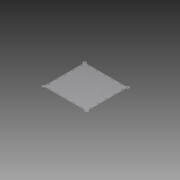
# Autodesk Inventor part: TopPlate2
Saved by Autodesk Inventor 2015 SP1 (Build 190203100, 203)
## iProperties
Created: 2014-08-06
Part Number: TopPlate2
Material: Acrylic, Clear
Document SubType Name: Modeling
Designer: Patrick Camilleri
Density: 1.19 g/cm^3
Appearance: Transparent - Clear
Mass: 654.149 g
Surface Area: 1962.87 cm^2
Volume: 549.705 cm^3
Author: Patrick Camilleri
Autodesk Inventor part; units mm, degrees
note: some values were not read from the file. Chosen so that the rebuilt part matches the saved one: direction of "Emboss9".
ref_plane "YZ Plane" through (0, 0, 0) normal (1, 0, 0) x (0, 1, 0)
ref_plane "XZ Plane" through (0, 0, 0) normal (0, 1, 0) x (-1, 0, 0)
sketch "Sketch1" plane through (0, 0, 0) normal (0, 0, 1) x (1, 0, 0)
  line L0 (-177, -128) -> (92, -128)
  line L1 (92, -128) -> (92, 128)
  line L2 (92, 128) -> (-177, 128)
  line L3 (-177, 128) -> (-177, -128)
  line L4 (-177, 0) -> (92, 0) construction
  line L5 (0, -128) -> (0, 128) construction
  point P0 (0, 0)
  point P1 (0, 0)
  dimension "d160" = 256
  dimension "d161" = 177
  dimension "d162" = 92
  constraints: 12 end point, 3 midpoint, 2 parallel, 2 perpendicular, 2 point on line, 1 coincident, 1 horizontal
  measures "d160" distance of L0.end L1.end
  measures "d161" distance between parallel lines of L3 L5
  measures "d162" distance between parallel lines of L1 L5
extrude "Extrusion1" add sketch "Sketch1" along normal blind 5
sketch "Sketch2" plane through (0, 0, 5) normal (0, 0, 1) x (1, 0, 0)
  line L0 (-172.1, 7.475) -> (-168.9, 7.475)
  line L1 (-168.9, 7.475) -> (-168.9, -7.475)
  line L2 (-168.9, -7.475) -> (-172.1, -7.475)
  line L3 (-172.1, -7.475) -> (-172.1, 7.475)
  line L4 (-172.1, 7.475) -> (-168.9, -7.475) construction
  line L5 (-168.9, 7.475) -> (-172.1, -7.475) construction
  line L6 (-177, -128) -> (92, -128) projected
  line L7 (92, -128) -> (92, 128) projected
  line L8 (92, 128) -> (-177, 128) projected
  line L9 (-177, 128) -> (-177, -128) projected
  line L10 (83.9, -7.475) -> (87.1, -7.475)
  line L11 (87.1, -7.475) -> (87.1, 7.475)
  line L12 (87.1, 7.475) -> (83.9, 7.475)
  line L13 (83.9, 7.475) -> (83.9, -7.475)
  line L14 (83.9, -7.475) -> (87.1, 7.475) construction
  line L15 (87.1, -7.475) -> (83.9, 7.475) construction
  line L16 (-170.5, -121.5) -> (85.5, -121.5) construction
  line L17 (85.5, -121.5) -> (85.5, 121.5) construction
  line L18 (85.5, 121.5) -> (-170.5, 121.5) construction
  line L19 (-170.5, 121.5) -> (-170.5, -121.5) construction
  point P0 (0, 0)
  point P1 (-170.5, 0)
  point P2 (85.5, 0)
  point P3 (85.5, 0)
  point P4 (-170.5, 0)
  dimension "d77" = 3.2
  dimension "d78" = 14.95
  dimension "d163" = 3.2
  dimension "d164" = 14.95
  dimension "d187" = 6.5
  constraints: 32 end point, 8 midpoint, 4 parallel, 2 horizontal, 2 perpendicular, 3 other
  measures "d77" distance of L1.end L2.end
  measures "d78" distance of L0.end L1.end
  measures "d163" distance of L12.end L11.end
  measures "d164" distance of L11.end L10.end
  measures "d187" distance between parallel lines of L9 L19
extrude "Extrusion3" cut sketch "Sketch2" against normal through all contours L0 L1 L2 L3 | L13 L12 L11 L10
sketch "Sketch3" plane through (0, 0, 5) normal (0, 0, 1) x (1, 0, 0)
  line L0 (-152.475, 123.1) -> (-137.525, 123.1)
  line L1 (-137.525, 123.1) -> (-137.525, 119.9)
  line L2 (-137.525, 119.9) -> (-152.475, 119.9)
  line L3 (-152.475, 119.9) -> (-152.475, 123.1)
  line L4 (-152.475, 123.1) -> (-137.525, 119.9) construction
  line L5 (-137.525, 123.1) -> (-152.475, 119.9) construction
  line L6 (-152.475, -119.9) -> (-137.525, -119.9)
  line L7 (-137.525, -119.9) -> (-137.525, -123.1)
  line L8 (-137.525, -123.1) -> (-152.475, -123.1)
  line L9 (-152.475, -123.1) -> (-152.475, -119.9)
  line L10 (-152.475, -119.9) -> (-137.525, -123.1) construction
  line L11 (-137.525, -119.9) -> (-152.475, -123.1) construction
  line L12 (-172.1, -7.475) -> (-172.1, 7.475) projected
  line L13 (-172.1, 7.475) -> (-168.9, 7.475) projected
  line L14 (-168.9, 7.475) -> (-168.9, -7.475) projected
  line L15 (-168.9, -7.475) -> (-172.1, -7.475) projected
  line L16 (-177, -128) -> (92, -128) projected
  line L17 (92, 128) -> (-177, 128) projected
  line L18 (-177, 128) -> (-177, -128) projected
  point P0 (0, 0)
  point P1 (-145, 121.5)
  point P2 (-145, -121.5)
  dimension "d125" = 14.95
  dimension "d126" = 3.2
  dimension "d128" = 14.95
  dimension "d129" = 3.2
  dimension "d198" = 32
  dimension "d199" = 6.5
  dimension "d200" = 32
  dimension "d201" = 6.5
  constraints: 24 end point, 4 midpoint, 4 parallel, 2 horizontal, 2 perpendicular
  measures "d125" distance of L1.end L2.end
  measures "d126" distance of L0.end L1.end
  measures "d128" distance of L7.end L8.end
  measures "d129" distance of L6.end L7.end
  measures "d198" distance from line of L18 point (-145, 121.5)
  measures "d199" distance from line of L17 point (-145, 121.5)
  measures "d200" distance from line of L18 point (-145, -121.5)
  measures "d201" distance from line of L16 point (-145, -121.5)
extrude "Extrusion4" cut sketch "Sketch3" against normal through all contours L0 L1 L2 L3 | L6 L7 L8 L9
pattern_linear "Rectangular Pattern1" count 5 spacing 50 along (1, 0, 0) of "Extrusion4"
pattern_linear "Rectangular Pattern2" count 5 spacing 50 along (0, -1, 0) of "Extrusion3" first direction both ways yes
sketch "Sketch7" plane through (0, 0, 5) normal (0, 0, 1) x (1, 0, 0)
  circle A0 centre (-177, -128) radius 10
  circle A1 centre (92, -128) radius 10
  point P0 (0, 0)
  dimension "d165" = 20
  dimension "d166" = 20
  constraints: 2 centre point, 2 coincident
  measures "d165" diameter of A0
  measures "d166" diameter of A1
extrude "Extrusion6" add sketch "Sketch7" against normal blind 5
mirror "Mirror7" about plane through (0, 0, 0) normal (0, 1, 0) of "Extrusion6"
hole "Hole6" at (-177, -128, 5) direction (0, 0, -1) diameter 6 end through all
hole "Hole7" at (92, -128, 5) direction (0, 0, -1) diameter 6 end through all
mirror "Mirror8" about plane through (0, 0, 0) normal (0, 1, 0) of "Hole6", "Hole7"
sketch "Sketch9" plane through (0, 0, 5) normal (0, 0, 1) x (1, 0, 0)
  line L0 (-168.9, 7.475) -> (-168.9, -7.475) projected
  line L1 (53.25, 2.425) -> (58.2, 2.425)
  line L2 (58.2, 2.425) -> (58.2, -2.425)
  line L3 (58.2, -2.425) -> (53.25, -2.425)
  line L4 (53.25, -2.425) -> (53.25, 2.425)
  point P0 (0, 0)
  point P1 (53.25, 0)
  point P2 (53.25, 0)
  dimension "d193" = 222.15
  dimension "d194" = 4.95
  dimension "d195" = 4.85
  constraints: 8 end point, 2 parallel, 1 coincident, 1 horizontal, 1 midpoint, 1 perpendicular
  measures "d193" distance from line of point (53.25, 0) L0
  measures "d194" distance of L2.end L3.end
  measures "d195" distance of L1.end L2.end
extrude "SquareHole" cut sketch "Sketch9" against normal through all
ref_plane "Logo Work Plane" through (0, 0, 0) normal (0, 0, 1) x (1, 0, 0)
sketch "Sail" plane through (0, 0, 0) normal (0, 0, 1) x (1, 0, 0)
  spline S0 degree 3 poles (-23.7243, -21.4525) (-16.5615, -20.6314) (-13.4344, -21.4525) (-13.1432, -24.6262) knots 0 0 0 0 1 1 1 1
  line L0 (-23.7243, -21.4525) -> (-16.5615, -20.6314) construction
  line L1 (-16.5615, -20.6314) -> (-13.4344, -21.4525) construction
  line L2 (-13.4344, -21.4525) -> (-13.1432, -24.6262) construction
  spline S1 degree 3 poles (-13.1432, -24.6262) (-10.2911, -18.8934) (2.9582, 7.7384) (-29.3731, 27.8226) knots 1 1 1 1 2 2 2 2
  line L3 (-13.1432, -24.6262) -> (-10.2911, -18.8934) construction
  line L4 (-10.2911, -18.8934) -> (2.9582, 7.7384) construction
  line L5 (2.9582, 7.7384) -> (-29.3731, 27.8226) construction
  spline S2 degree 3 poles (-29.3731, 27.8226) (-31.8581, 29.0036) (-47.8295, 36.594) (-77.3586, 36.594) knots 2 2 2 2 3 3 3 3
  line L6 (-29.3731, 27.8226) -> (-31.8581, 29.0036) construction
  line L7 (-31.8581, 29.0036) -> (-47.8295, 36.594) construction
  line L8 (-47.8295, 36.594) -> (-77.3586, 36.594) construction
  spline S3 degree 3 poles (-77.3586, 36.594) (-70.2712, 34.7172) (-49.772, 21.1687) (-66.3123, -37.5545) knots 3 3 3 3 4 4 4 4
  line L9 (-77.3586, 36.594) -> (-70.2712, 34.7172) construction
  line L10 (-70.2712, 34.7172) -> (-49.772, 21.1687) construction
  line L11 (-49.772, 21.1687) -> (-66.3123, -37.5545) construction
  spline S4 degree 3 poles (-66.3123, -37.5545) (-66.2924, -37.5407) (-46.3945, -23.7631) (-23.7243, -21.4525) knots 4 4 4 4 5 5 5 5
  line L12 (-66.3123, -37.5545) -> (-46.3945, -23.7631) construction
  line L13 (-46.3945, -23.7631) -> (-23.7243, -21.4525) construction
  line L14 (-25.8335, -22.8285) -> (-27.8287, -31.4427)
  spline S5 degree 3 poles (-27.8287, -31.4427) (-27.7953, -31.4332) (-14.6395, -28.1149) (-12.2292, -25.2426) knots 0 0 0 0 1 1 1 1
  line L15 (-27.8287, -31.4427) -> (-27.7953, -31.4332) construction
  line L16 (-27.7953, -31.4332) -> (-14.6395, -28.1149) construction
  line L17 (-14.6395, -28.1149) -> (-12.2292, -25.2426) construction
  spline S6 degree 3 poles (-12.2292, -25.2426) (-12.2293, -25.2425) (7.7964, 7.1612) (-28.8599, 29.1216) knots 1 1 1 1 2 2 2 2
  line L18 (-12.2292, -25.2426) -> (-12.2293, -25.2425) construction
  line L19 (-12.2293, -25.2425) -> (7.7964, 7.1612) construction
  line L20 (7.7964, 7.1612) -> (-28.8599, 29.1216) construction
  spline S7 degree 3 poles (-28.8599, 29.1216) (-28.9152, 29.1547) (-47.9851, 39.8143) (-82.821, 37.2661) knots 2 2 2 2 3 3 3 3
  line L21 (-28.8599, 29.1216) -> (-28.9152, 29.1547) construction
  line L22 (-28.9152, 29.1547) -> (-47.9851, 39.8143) construction
  line L23 (-47.9851, 39.8143) -> (-82.821, 37.2661) construction
  spline S8 degree 3 poles (-82.821, 37.2661) (-81.9776, 37.033) (-46.5816, 35.4518) (-68.4927, -40.1633) knots 3 3 3 3 4 4 4 4
  line L24 (-82.821, 37.2661) -> (-81.9776, 37.033) construction
  line L25 (-81.9776, 37.033) -> (-46.5816, 35.4518) construction
  line L26 (-46.5816, 35.4518) -> (-68.4927, -40.1633) construction
  spline S9 degree 3 poles (-68.4927, -40.1633) (-67.9278, -39.7931) (-46.3371, -25.6429) (-25.8335, -22.8285) knots 4 4 4 4 5 5 5 5
  line L27 (-68.4927, -40.1633) -> (-67.9278, -39.7931) construction
  line L28 (-67.9278, -39.7931) -> (-46.3371, -25.6429) construction
  line L29 (-46.3371, -25.6429) -> (-25.8335, -22.8285) construction
  line L30 (-84.1279, 4.5809) -> (-64.8809, 4.5809) construction
  line L31 (-64.8809, 4.5809) -> (-64.8809, -10.2757) construction
  line L32 (-64.8809, -10.2757) -> (-84.1279, -10.2757) construction
  line L33 (-84.1279, -10.2757) -> (-84.1279, 4.5809) construction
  line L34 (-58.4488, 4.4304) -> (-7.0901, 4.4304) construction
  line L35 (-7.0901, 4.4304) -> (-7.0901, -11.2966) construction
  line L36 (-7.0901, -11.2966) -> (-58.4488, -11.2966) construction
  line L37 (-58.4488, -11.2966) -> (-58.4488, 4.4304) construction
  line L38 (-89.1022, -5.5775) -> (-1.5111, -5.5775) construction
  line L39 (-57.4656, -5.5696) -> (-57.4656, 4.4304)
  line L40 (-57.4656, 4.4304) -> (-55.6058, 4.4304)
  line L41 (-55.6058, 4.4304) -> (-51.7034, -2.2693)
  line L42 (-51.7034, -2.2693) -> (-51.7034, 4.4304)
  line L43 (-51.7034, 4.4304) -> (-49.9275, 4.4304)
  line L44 (-49.9275, 4.4304) -> (-49.9275, -5.5696)
  line L45 (-49.9275, -5.5696) -> (-51.8482, -5.5696)
  line L46 (-51.8482, -5.5696) -> (-55.6897, 0.9777)
  line L47 (-55.6897, 0.9777) -> (-55.6897, -5.5696)
  line L48 (-55.6897, -5.5696) -> (-57.4656, -5.5696)
  line L49 (-47.8848, -5.5696) -> (-47.8848, 4.4304)
  line L50 (-47.8848, 4.4304) -> (-46.025, 4.4304)
  line L51 (-46.025, 4.4304) -> (-42.1226, -2.2693)
  line L52 (-42.1226, -2.2693) -> (-42.1226, 4.4304)
  line L53 (-42.1226, 4.4304) -> (-40.3467, 4.4304)
  line L54 (-40.3467, 4.4304) -> (-40.3467, -5.5696)
  line L55 (-40.3467, -5.5696) -> (-42.2674, -5.5696)
  line L56 (-42.2674, -5.5696) -> (-46.1089, 0.9777)
  line L57 (-46.1089, 0.9777) -> (-46.1089, -5.5696)
  line L58 (-46.1089, -5.5696) -> (-47.8848, -5.5696)
  line L59 (-36.9702, -0.5315) -> (-38.6241, -0.219)
  spline S10 degree 2 poles (-38.6241, -0.219) (-38.3421, 0.8329) (-36.9854, 1.839) (-35.6439, 1.839) knots 0 0 0 1 2 2 2
  spline S11 degree 2 poles (-35.6439, 1.839) (-34.4244, 1.839) (-33.2354, 1.2292) (-32.7476, 0.2993) (-32.7476, -0.9507) knots 0 0 0 1 2 3 3 3
  line L60 (-32.7476, -0.9507) -> (-32.7705, -3.1915)
  spline S12 degree 2 poles (-32.7705, -3.1915) (-32.7705, -4.1443) (-32.5952, -5.0513) (-32.3589, -5.5696) knots 0 0 0 1 2 2 2
  line L61 (-32.3589, -5.5696) -> (-34.1577, -5.5696)
  spline S13 degree 2 poles (-34.1577, -5.5696) (-34.2263, -5.379) (-34.333, -5.0056) knots 0 0 0 1 1 1
  spline S14 degree 2 poles (-34.333, -5.0056) (-34.3787, -4.8303) (-34.3939, -4.7769) knots 0 0 0 1 1 1
  spline S15 degree 2 poles (-34.3939, -4.7769) (-34.8665, -5.2495) (-35.926, -5.7296) (-36.5281, -5.7296) knots 0 0 0 1 2 2 2
  spline S16 degree 2 poles (-36.5281, -5.7296) (-37.5875, -5.7296) (-38.8147, -4.5178) (-38.8147, -3.5879) knots 0 0 0 1 2 2 2
  spline S17 degree 2 poles (-38.8147, -3.5879) (-38.8147, -2.9705) (-38.2583, -2.0101) (-37.2522, -1.4995) (-36.307, -1.3089) knots 0 0 0 1 2 3 3 3
  spline S18 degree 2 poles (-36.307, -1.3089) (-35.0342, -1.0574) (-34.5388, -0.8364) knots 0 0 0 1 1 1
  line L62 (-34.5388, -0.8364) -> (-34.5388, -0.6458)
  spline S19 degree 2 poles (-34.5388, -0.6458) (-34.5388, -0.097) (-35.057, 0.3755) (-35.7735, 0.3755) knots 0 0 0 1 2 2 2
  spline S20 degree 2 poles (-35.7735, 0.3755) (-36.2613, 0.3755) (-36.8025, -0.0284) (-36.9702, -0.5315) knots 0 0 0 1 2 2 2
  spline S21 degree 2 poles (-34.5388, -2.0864) (-34.8894, -2.2083) (-36.4061, -2.5513) (-36.6348, -2.7114) knots 0 0 0 1 2 2 2
  spline S22 degree 2 poles (-36.6348, -2.7114) (-36.993, -2.9781) (-36.993, -3.3897) knots 0 0 0 1 1 1
  spline S23 degree 2 poles (-36.993, -3.3897) (-36.993, -3.7937) (-36.4214, -4.3806) (-35.9793, -4.3806) knots 0 0 0 1 2 2 2
  spline S24 degree 2 poles (-35.9793, -4.3806) (-35.4915, -4.3806) (-35.0418, -4.0376) knots 0 0 0 1 1 1
  spline S25 degree 2 poles (-35.0418, -4.0376) (-34.7141, -3.7784) (-34.6074, -3.405) knots 0 0 0 1 1 1
  spline S26 degree 2 poles (-34.6074, -3.405) (-34.5388, -3.161) (-34.5388, -2.4675) knots 0 0 0 1 1 1
  line L63 (-34.5388, -2.4675) -> (-34.5388, -2.0864)
  line L64 (-31.025, -5.5696) -> (-31.025, 4.4304)
  line L65 (-31.025, 4.4304) -> (-29.2034, 4.4304)
  line L66 (-29.2034, 4.4304) -> (-29.2034, -0.8745)
  line L67 (-29.2034, -0.8745) -> (-27.0692, 1.6789)
  line L68 (-27.0692, 1.6789) -> (-24.8284, 1.6789)
  line L69 (-24.8284, 1.6789) -> (-27.1836, -0.9659)
  line L70 (-27.1836, -0.9659) -> (-24.6607, -5.5696)
  line L71 (-24.6607, -5.5696) -> (-26.6272, -5.5696)
  line L72 (-26.6272, -5.5696) -> (-28.3574, -2.3074)
  line L73 (-28.3574, -2.3074) -> (-29.2034, -3.2525)
  line L74 (-29.2034, -3.2525) -> (-29.2034, -5.5696)
  line L75 (-29.2034, -5.5696) -> (-31.025, -5.5696)
  line L76 (-19.5997, -3.2601) -> (-17.7857, -3.5803)
  spline S27 degree 2 poles (-17.7857, -3.5803) (-18.1363, -4.6321) (-19.6455, -5.7296) (-20.7735, -5.7296) knots 0 0 0 1 2 2 2
  spline S28 degree 2 poles (-20.7735, -5.7296) (-22.5723, -5.7296) (-23.4336, -4.4949) knots 0 0 0 1 1 1
  spline S29 degree 2 poles (-23.4336, -4.4949) (-24.1119, -3.504) (-24.1119, -2.0025) knots 0 0 0 1 1 1
  spline S30 degree 2 poles (-24.1119, -2.0025) (-24.1119, -0.1961) (-22.3208, 1.839) (-20.9564, 1.839) knots 0 0 0 1 2 2 2
  spline S31 degree 2 poles (-20.9564, 1.839) (-19.4244, 1.839) (-17.6485, -0.2952) (-17.6866, -2.4979) knots 0 0 0 1 2 2 2
  line L77 (-17.6866, -2.4979) -> (-22.2445, -2.4979)
  spline S32 degree 2 poles (-22.2445, -2.4979) (-22.2217, -3.3516) (-21.3833, -4.2967) (-20.7583, -4.2967) knots 0 0 0 1 2 2 2
  spline S33 degree 2 poles (-20.7583, -4.2967) (-20.3314, -4.2967) (-19.7522, -3.8089) (-19.5997, -3.2601) knots 0 0 0 1 2 2 2
  spline S34 degree 2 poles (-19.493, -1.3242) (-19.5159, -0.4934) (-20.2857, 0.3755) (-20.8497, 0.3755) knots 0 0 0 1 2 2 2
  spline S35 degree 2 poles (-20.8497, 0.3755) (-21.4442, 0.3755) (-21.833, -0.0818) knots 0 0 0 1 1 1
  spline S36 degree 2 poles (-21.833, -0.0818) (-22.2217, -0.5391) (-22.2141, -1.3242) knots 0 0 0 1 1 1
  line L78 (-22.2141, -1.3242) -> (-19.493, -1.3242)
  line L79 (-14.4549, -5.5696) -> (-16.2766, -5.5696)
  line L80 (-16.2766, -5.5696) -> (-16.2766, 1.6789)
  line L81 (-16.2766, 1.6789) -> (-14.5845, 1.6789)
  line L82 (-14.5845, 1.6789) -> (-14.5845, 0.6499)
  spline S37 degree 2 poles (-14.5845, 0.6499) (-14.15, 1.3816) (-13.4564, 1.839) (-13.0144, 1.839) knots 0 0 0 1 2 2 2
  spline S38 degree 2 poles (-13.0144, 1.839) (-12.397, 1.839) (-11.8177, 1.4731) knots 0 0 0 1 1 1
  line L83 (-11.8177, 1.4731) -> (-12.3741, -0.1961)
  spline S39 degree 2 poles (-12.3741, -0.1961) (-12.8391, 0.1164) (-13.2354, 0.1164) knots 0 0 0 1 1 1
  spline S40 degree 2 poles (-13.2354, 0.1164) (-13.6165, 0.1164) (-14.15, -0.3257) (-14.4549, -1.4842) (-14.4549, -3.3364) knots 0 0 0 1 2 3 3 3
  line L84 (-14.4549, -3.3364) -> (-14.4549, -5.5696)
  line L85 (-83.6477, -2.3246) -> (-81.7803, -2.134)
  spline S41 degree 2 poles (-81.7803, -2.134) (-81.6127, -3.1249) (-80.5837, -4.0548) (-79.7072, -4.0548) knots 0 0 0 1 2 2 2
  spline S42 degree 2 poles (-79.7072, -4.0548) (-78.7849, -4.0548) (-77.8474, -3.2316) (-77.8474, -2.6752) knots 0 0 0 1 2 2 2
  spline S43 degree 2 poles (-77.8474, -2.6752) (-77.8474, -2.317) (-78.2438, -1.8215) (-78.7316, -1.6386) knots 0 0 0 1 2 2 2
  spline S44 degree 2 poles (-78.7316, -1.6386) (-79.0746, -1.5167) (-80.2712, -1.2042) knots 0 0 0 1 1 1
  spline S45 degree 2 poles (-80.2712, -1.2042) (-81.8108, -0.8002) (-82.4282, -0.2133) knots 0 0 0 1 1 1
  spline S46 degree 2 poles (-82.4282, -0.2133) (-83.3047, 0.6099) (-83.3047, 1.7913) knots 0 0 0 1 1 1
  spline S47 degree 2 poles (-83.3047, 1.7913) (-83.3047, 2.5611) (-82.4816, 3.8873) (-80.9343, 4.5809) (-79.8367, 4.5809) knots 0 0 0 1 2 3 3 3
  spline S48 degree 2 poles (-79.8367, 4.5809) (-78.0532, 4.5809) (-76.2468, 2.9345) (-76.2011, 1.555) knots 0 0 0 1 2 2 2
  line L86 (-76.2011, 1.555) -> (-78.1218, 1.4635)
  spline S49 degree 2 poles (-78.1218, 1.4635) (-78.2438, 2.2333) (-79.0517, 2.9117) (-79.8596, 2.9117) knots 0 0 0 1 2 2 2
  spline S50 degree 2 poles (-79.8596, 2.9117) (-80.6904, 2.9117) (-81.163, 2.5535) knots 0 0 0 1 1 1
  spline S51 degree 2 poles (-81.163, 2.5535) (-81.4678, 2.3172) (-81.4678, 1.9285) knots 0 0 0 1 1 1
  spline S52 degree 2 poles (-81.4678, 1.9285) (-81.4678, 1.5778) (-81.1858, 1.3187) knots 0 0 0 1 1 1
  spline S53 degree 2 poles (-81.1858, 1.3187) (-80.82, 0.9986) (-78.0227, 0.305) (-76.6813, -0.4344) (-75.9267, -1.7225) (-75.9267, -2.6752) knots 0 0 0 1 2 3 4 4 4
  spline S54 degree 2 poles (-75.9267, -2.6752) (-75.9267, -3.5289) (-76.8337, -5.0304) (-78.4953, -5.7621) (-79.73, -5.7621) knots 0 0 0 1 2 3 3 3
  spline S55 degree 2 poles (-79.73, -5.7621) (-81.5288, -5.7621) (-83.4572, -4.009) (-83.6477, -2.3246) knots 0 0 0 1 2 2 2
  line L87 (-74.3794, 1.6617) -> (-72.6797, 1.6617)
  line L88 (-72.6797, 1.6617) -> (-72.6797, 0.5946)
  spline S56 degree 2 poles (-72.6797, 0.5946) (-72.352, 1.1434) (-71.2239, 1.8217) (-70.538, 1.8217) knots 0 0 0 1 2 2 2
  spline S57 degree 2 poles (-70.538, 1.8217) (-69.3337, 1.8217) (-67.6645, -0.1523) (-67.6645, -1.9206) knots 0 0 0 1 2 2 2
  spline S58 degree 2 poles (-67.6645, -1.9206) (-67.6645, -3.7347) (-69.3489, -5.7469) (-70.5456, -5.7469) knots 0 0 0 1 2 2 2
  spline S59 degree 2 poles (-70.5456, -5.7469) (-71.1172, -5.7469) (-72.0471, -5.2667) (-72.5578, -4.6874) knots 0 0 0 1 2 2 2
  line L89 (-72.5578, -4.6874) -> (-72.5578, -8.3459)
  line L90 (-72.5578, -8.3459) -> (-74.3794, -8.3459)
  line L91 (-74.3794, -8.3459) -> (-74.3794, 1.6617)
  spline S60 degree 2 poles (-72.5806, -1.8368) (-72.5806, -3.0563) (-71.6584, -4.2225) (-70.9953, -4.2225) knots 0 0 0 1 2 2 2
  spline S61 degree 2 poles (-70.9953, -4.2225) (-70.3627, -4.2225) (-69.5166, -3.1554) (-69.5166, -1.9359) knots 0 0 0 1 2 2 2
  spline S62 degree 2 poles (-69.5166, -1.9359) (-69.5166, -0.8002) (-70.3855, 0.305) (-71.0258, 0.305) knots 0 0 0 1 2 2 2
  spline S63 degree 2 poles (-71.0258, 0.305) (-71.6965, 0.305) (-72.5806, -0.7773) (-72.5806, -1.8368) knots 0 0 0 1 2 2 2
  line L92 (-66.2239, -5.5868) -> (-66.2239, 1.6617)
  line L93 (-66.2239, 1.6617) -> (-64.4023, 1.6617)
  line L94 (-64.4023, 1.6617) -> (-64.4023, -5.5868)
  line L95 (-64.4023, -5.5868) -> (-66.2239, -5.5868)
  line L96 (-66.2239, 2.6373) -> (-66.2239, 4.4132)
  line L97 (-66.2239, 4.4132) -> (-64.4023, 4.4132)
  line L98 (-64.4023, 4.4132) -> (-64.4023, 2.6373)
  line L99 (-64.4023, 2.6373) -> (-66.2239, 2.6373)
  point P0 (0, 0)
  constraints: 5 end point, 2 coincident, 2 point on line, 1 horizontal, 35 other
emboss "Emboss9" sketch "Sail" operation add depth 1 direction (0, 0, 1)
equation "\"d166\" = d165"
equation "\"kerf\" = 0.15"
equation "\"slot_w\" = 3.35"
equation "\"slot_l\" = 15.1"
body "Solid1"
